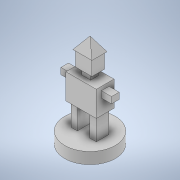
# Autodesk Inventor part: Vasile5-6Bridge.stl
Saved by Autodesk Inventor 2020 (Build 240168000, 168)
## iProperties
Created: 2020-03-17
Part Number: Vasile5-6Bridge.stl
Material: Generic
Document SubType Name: Modeling
Designer: al
Density: 1 g/cm^3
Appearance: Default
Author: al
Autodesk Inventor part; units mm, degrees
ref_plane "YZ Plane" through (0, 0, 0) normal (1, 0, 0) x (0, 1, 0)
ref_plane "XZ Plane" through (0, 0, 0) normal (0, 1, 0) x (-1, 0, 0)
ref_plane "XY Plane" through (0, 0, 0) normal (0, 0, 1) x (1, 0, 0)
sketch "Sketch1" plane through (0, 0, 0) normal (0, 0, 1) x (1, 0, 0)
  circle A0 centre (0, 0) radius 25.4
  dimension "d0" = 50.8
  constraints: 1 centre point, 1 coincident
  measures "d0" diameter of A0
extrude "Extrusion1" add sketch "Sketch1" along normal blind 11.43
sketch "Sketch2" plane through (0, 0, 11.43) normal (0, 0, 1) x (1, 0, 0)
  line L0 (0, 0) -> (-6.35, 0)
  line L1 (0, 0) -> (6.35, 0)
  line L2 (-6.35, 0) -> (-6.35, 6.35)
  line L3 (-6.35, 6.35) -> (-12.7, 6.35)
  line L4 (-12.7, 6.35) -> (-12.7, -6.35)
  line L5 (-12.7, -6.35) -> (-6.35, -6.35)
  line L6 (-6.35, -6.35) -> (-6.35, 0)
  line L7 (6.35, 0) -> (6.35, 6.35)
  line L8 (6.35, 6.35) -> (12.7, 6.35)
  line L9 (12.7, 6.35) -> (12.7, -6.35)
  line L10 (12.7, -6.35) -> (6.35, -6.35)
  line L11 (6.35, -6.35) -> (6.35, 0)
  dimension "d3" = 6.35
  dimension "d4" = 6.35
  dimension "d5" = 6.35
  dimension "d6" = 6.35
  dimension "d7" = 12.7
  dimension "d8" = 6.35
  dimension "d9" = 6.35
  dimension "d10" = 12.7
  constraints: 24 end point, 5 perpendicular, 4 horizontal, 2 vertical, 1 collinear, 1 point on line
  measures "d3" distance of L0.start L0.end
  measures "d4" distance of L0.start L1.end
  measures "d5" distance of L0.end L2.end
  measures "d6" distance of L2.end L3.end
  measures "d7" distance of L3.end L4.end
  measures "d8" distance of L1.end L7.end
  measures "d9" distance of L7.end L8.end
  measures "d10" distance of L8.end L9.end
extrude "Extrusion2" add sketch "Sketch2" along normal blind 22.86
sketch "Sketch3" plane through (0, 0, 34.29) normal (0, 0, 1) x (1, 0, 0)
  line L0 (-12.7, 6.35) -> (-12.7, -6.35) projected
  line L1 (-12.7, -6.35) -> (-12.7, -8.89)
  line L2 (-12.7, -8.89) -> (-15.24, -8.89)
  line L3 (-15.24, -8.89) -> (15.24, -8.89)
  line L4 (15.24, -8.89) -> (15.24, 8.89)
  line L5 (15.24, 8.89) -> (-15.24, 8.89)
  line L6 (-15.24, 8.89) -> (-15.24, -8.89)
  point P0 (0, 0)
  dimension "d13" = 2.54
  dimension "d14" = 2.54
  dimension "d15" = 30.48
  dimension "d16" = 17.78
  constraints: 12 end point, 2 parallel, 2 perpendicular, 1 horizontal, 1 vertical
  measures "d13" distance of L0.end L1.end
  measures "d14" distance of L1.end L2.end
  measures "d15" distance of L5.end L4.end
  measures "d16" distance of L4.end L3.end
extrude "Extrusion3" add sketch "Sketch3" along normal blind 25.4
sketch "Sketch4" plane through (-15.24, -8.89, 34.29) normal (-1, 0, 0) x (0, 0, 1)
  line L0 (0, 17.78) -> (25.4, 17.78) projected
  line L1 (0, 17.78) -> (0, 12.7)
  line L2 (0, 0) -> (0, 17.78) projected
  line L3 (0, 12.7) -> (15.24, 12.7)
  line L4 (15.24, 12.7) -> (15.24, 5.08)
  line L5 (15.24, 5.08) -> (21.59, 5.08)
  line L6 (21.59, 5.08) -> (21.59, 12.7)
  line L7 (21.59, 12.7) -> (15.24, 12.7)
  point P0 (-34.29, 8.89)
  dimension "d19" = 5.08
  dimension "d20" = 15.24
  dimension "d21" = 7.62
  dimension "d22" = 6.35
  dimension "d23" = 7.62
  constraints: 12 end point, 2 horizontal, 2 perpendicular, 1 point on line
  measures "d19" distance of L0.start L1.end
  measures "d20" distance of L1.end L3.end
  measures "d21" distance of L3.end L4.end
  measures "d22" distance of L4.end L5.end
  measures "d23" distance of L5.end L6.end
extrude "Extrusion4" add sketch "Sketch4" along normal blind 10.16
sketch "Sketch5" plane through (15.24, -8.89, 34.29) normal (1, 0, 0) x (0, 0, -1)
  line L0 (0, 0) -> (0, 5.08)
  line L1 (0, 17.78) -> (0, 0) projected
  line L2 (0, 5.08) -> (-15.24, 5.08)
  line L3 (-15.24, 5.08) -> (-21.59, 5.08)
  line L4 (-21.59, 5.08) -> (-21.59, 12.7)
  line L5 (-21.59, 12.7) -> (-15.24, 12.7)
  line L6 (-15.24, 12.7) -> (-15.24, 5.08)
  point P0 (34.29, 8.89)
  dimension "d26" = 5.08
  dimension "d27" = 15.24
  dimension "d28" = 6.35
  dimension "d29" = 7.62
  constraints: 12 end point, 2 parallel, 2 perpendicular, 1 horizontal, 1 point on line
  measures "d26" distance of L0.start L0.end
  measures "d27" distance of L0.end L2.end
  measures "d28" distance of L4.end L5.end
  measures "d29" distance of L3.end L4.end
extrude "Extrusion5" add sketch "Sketch5" along normal blind 10.16
sketch "Sketch6" plane through (0, 0, 59.69) normal (0, 0, 1) x (1, 0, 0)
  line L0 (-15.24, -8.89) -> (15.24, -8.89) projected
  line L1 (15.24, -8.89) -> (4.445, -8.89)
  line L2 (-15.24, 8.89) -> (-15.24, -8.89) projected
  line L3 (-15.24, -8.89) -> (-4.445, -8.89)
  line L4 (-4.445, -8.89) -> (-4.445, -3.81)
  line L5 (15.24, 8.89) -> (-15.24, 8.89) projected
  line L6 (-4.445, -3.81) -> (4.445, -3.81)
  line L7 (4.445, -3.81) -> (4.445, 3.81)
  line L8 (4.445, 3.81) -> (-4.445, 3.81)
  line L9 (-4.445, 3.81) -> (-4.445, -3.81)
  point P0 (0, 0)
  dimension "d32" = 10.795
  dimension "d33" = 10.795
  dimension "d34" = 5.08
  dimension "d35" = 7.62
  constraints: 14 end point, 2 parallel, 2 perpendicular, 2 point on line, 1 horizontal
  measures "d32" distance of L0.end L1.end
  measures "d33" distance of L0.start L3.end
  measures "d34" distance of L3.end L4.end
  measures "d35" distance of L7.end L6.end
extrude "Extrusion6" add sketch "Sketch6" along normal blind 6.35
sketch "Sketch7" plane through (0, 0, 66.04) normal (0, 0, 1) x (1, 0, 0)
  line L0 (4.445, 3.81) -> (4.445, -3.81) projected
  line L1 (4.445, 3.81) -> (8.255, 3.81)
  line L2 (8.255, 3.81) -> (8.255, 6.35)
  line L3 (12.7, 6.35) -> (6.35, 6.35) projected
  line L4 (-12.7, -6.35) -> (-6.35, -6.35) projected
  line L5 (8.255, 6.35) -> (-8.255, 6.35)
  line L6 (-8.255, 6.35) -> (-8.255, -6.35)
  line L7 (-8.255, -6.35) -> (8.255, -6.35)
  line L8 (8.255, -6.35) -> (8.255, 6.35)
  point P0 (0, 0)
  dimension "d38" = 3.81
  dimension "d39" = 16.51
  constraints: 12 end point, 2 horizontal, 2 parallel, 2 perpendicular, 2 point on line
  measures "d38" distance of L0.start L1.end
  measures "d39" distance of L7.end L6.end
extrude "Extrusion7" add sketch "Sketch7" along normal blind 15.24
sketch "Sketch8" plane through (0, 0, 81.28) normal (0, 0, 1) x (1, 0, 0)
  line L0 (-8.255, 6.35) -> (-8.255, -6.35) projected
  line L1 (-8.255, -6.35) -> (-8.255, -7.62)
  line L2 (-8.255, -7.62) -> (-9.525, -7.62)
  line L3 (-9.525, -7.62) -> (9.525, -7.62)
  line L4 (9.525, -7.62) -> (9.525, 7.62)
  line L5 (9.525, 7.62) -> (-9.525, 7.62)
  line L6 (-9.525, 7.62) -> (-9.525, -7.62)
  point P0 (0, 0)
  dimension "d42" = 1.27
  dimension "d43" = 1.27
  dimension "d44" = 15.24
  constraints: 12 end point, 2 parallel, 2 perpendicular, 1 horizontal, 1 vertical
  measures "d42" distance of L0.end L1.end
  measures "d43" distance of L1.end L2.end
  measures "d44" distance of L3.end L4.end
extrude "Extrusion8" add sketch "Sketch8" along normal blind 12.7
sketch "Sketch9" plane through (-9.525, 7.62, 81.28) normal (0, 1, 0) x (1, 0, 0)
  line L0 (19.05, 0) -> (0, 0) projected
  line L1 (19.05, 0) -> (19.05, -12.7)
  line L2 (19.05, -12.7) -> (9.525, -12.7)
  line L3 (19.05, -12.7) -> (0, -12.7) projected
  line L4 (9.525, -12.7) -> (19.05, 0)
  line L5 (9.525, -12.7) -> (0, -12.7)
  line L6 (0, 0) -> (0, -12.7) projected
  line L7 (0, 0) -> (0, -12.7)
  line L8 (9.525, -12.7) -> (0, 0)
  point P0 (9.525, 81.28)
  constraints: 12 end point, 2 vertical, 1 collinear, 1 midpoint
sketch "Sketch10" plane through (-9.525, -7.62, 81.28) normal (-1, 0, 0) x (0, 0, 1)
  line L0 (12.7, 0) -> (12.7, 15.24) projected
  line L1 (12.7, 15.24) -> (12.7, 7.62)
  line L2 (0, 0) -> (0, 15.24) projected
  line L3 (12.7, 7.62) -> (0, 15.24)
  line L4 (0, 15.24) -> (12.7, 15.24)
  line L5 (0, 0) -> (12.7, 0) projected
  line L6 (12.7, 0) -> (12.7, 7.62)
  line L7 (12.7, 7.62) -> (0, 0)
  line L8 (12.7, 0) -> (0, 0)
  point P0 (-81.28, 7.62)
  dimension "d47" = 7.62
  constraints: 12 end point, 2 perpendicular, 1 midpoint, 1 vertical
  measures "d47" distance of L0.end L1.end
extrude "Extrusion9" cut sketch "Sketch9" against normal blind 15.24 contours L1 L2 L4 | L8 L3 L6
extrude "Extrusion10" cut sketch "Sketch10" against normal blind 20.32 contours L5 L7 L0 | L3 L4 L0
body "Solid1"
